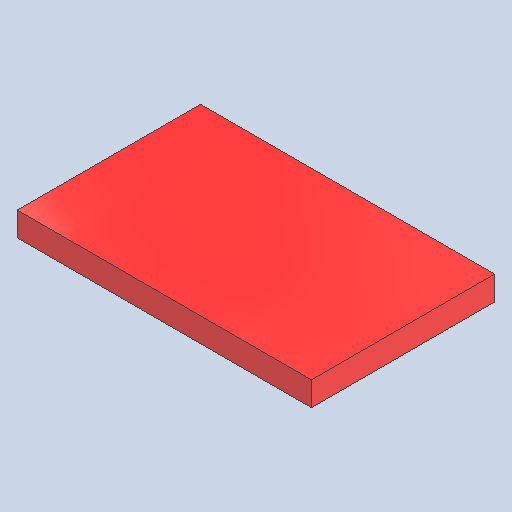
# Autodesk Inventor part: Battery
Saved by Autodesk Inventor 2025.2 (Build 292293000, 293)
## iProperties
Created: 2024-03-12
Part Number: Battery
Material: Generic
Document SubType Name: Modeling
Designer: mirun
Density: 1 g/cm^3
Appearance: Default
Author: mirun
Autodesk Inventor part; units mm, degrees
ref_plane "YZ Plane" through (0, 0, 0) normal (1, 0, 0) x (0, 1, 0)
ref_plane "XZ Plane" through (0, 0, 0) normal (0, 1, 0) x (-1, 0, 0)
ref_plane "XY Plane" through (0, 0, 0) normal (0, 0, 1) x (1, 0, 0)
sketch "Sketch1" plane through (0, 0, 0) normal (0, 1, 0) x (-1, 0, 0)
  line L0 (-30.5, 19) -> (30.5, 19)
  line L1 (30.5, 19) -> (30.5, -19)
  line L2 (30.5, -19) -> (-30.5, -19)
  line L3 (-30.5, -19) -> (-30.5, 19)
  line L4 (-30.5, 19) -> (30.5, -19) construction
  line L5 (30.5, 19) -> (-30.5, -19) construction
  point P0 (0, 0)
  dimension "d0" = 61
  dimension "d1" = 38
  constraints: 12 end point, 2 midpoint, 2 parallel, 1 horizontal, 1 perpendicular
  measures "d0" distance of L1.end L2.end
  measures "d1" distance of L0.end L1.end
extrude "Extrusion1" add sketch "Sketch1" along normal blind 5
body "Solid1"
